Autodesk Fusion 360 part; units mm, degrees
(part 3 of 5)
sketch "Rack Tooth" plane through (0, 7, 0) normal (0, 1, 0) x (-1, 0, 0)
  line L0 (-33, 45.0877) -> (-33, 8.0877) construction
  circle A0 centre (-25, 30) radius 8 construction
  line L1 (0, 30) -> (-50, 30) construction
  line L2 (-33, 30) -> (-27.4745, 14.8188) construction
  spline S0 degree 5 poles (-32.1641, 27.722) (-32.1682, 27.7207) (-32.1765, 27.7182) (-32.1891, 27.7148) (-32.206, 27.7109) (-32.2273, 27.707) (-32.2489, 27.7038) (-32.2705, 27.701) (-32.2923, 27.6984) (-32.3141, 27.696) (-32.3359, 27.6937) (-32.3578, 27.6917) (-32.3798, 27.6899) (-32.4018, 27.6885) (-32.4239, 27.6874) (-32.4461, 27.6866) (-32.4684, 27.686) (-32.4907, 27.6857) (-32.5131, 27.6856) (-32.5355, 27.6857) (-32.5579, 27.6859) (-32.5804, 27.6864) (-32.6029, 27.6871) (-32.6255, 27.6879) (-32.6481, 27.689) (-32.6708, 27.6903) (-32.6935, 27.6918) (-32.7162, 27.6934) (-32.7389, 27.6953) (-32.7617, 27.6973) (-32.7846, 27.6995) (-32.8074, 27.7018) (-32.8303, 27.7044) (-32.8532, 27.7071) (-32.8761, 27.71) (-32.8991, 27.713) (-32.9221, 27.7162) (-32.9451, 27.7196) (-32.9681, 27.7232) (-32.9912, 27.7269) (-33.0142, 27.7307) (-33.0373, 27.7348) (-33.0605, 27.7389) (-33.0836, 27.7433) (-33.1067, 27.7478) (-33.1299, 27.7524) (-33.1531, 27.7572) (-33.1763, 27.7622) (-33.1995, 27.7673) (-33.2227, 27.7725) (-33.246, 27.7779) (-33.2692, 27.7835) (-33.2925, 27.7892) (-33.3158, 27.795) (-33.3391, 27.801) (-33.3624, 27.8071) (-33.3857, 27.8134) (-33.409, 27.8198) (-33.4323, 27.8264) (-33.4557, 27.833) (-33.479, 27.8399) (-33.5023, 27.8469) (-33.5257, 27.854) (-33.549, 27.8612) (-33.5724, 27.8686) (-33.5958, 27.8762) (-33.6191, 27.8838) (-33.6425, 27.8916) (-33.6659, 27.8996) (-33.6892, 27.9076) (-33.7126, 27.9158) (-33.7313, 27.9225) (-33.7453, 27.9276) (-33.7547, 27.931) (-33.7594, 27.9327) knots 0 0 0 0 0 0 0.01428571 0.02857143 0.04285714 0.05714286 0.07142857 0.08571429 0.1 0.11428571 0.12857143 0.14285714 0.15714286 0.17142857 0.18571429 0.2 0.21428571 0.22857143 0.24285714 0.25714286 0.27142857 0.28571429 0.3 0.31428571 0.32857143 0.34285714 0.35714286 0.37142857 0.38571429 0.4 0.41428571 0.42857143 0.44285714 0.45714286 0.47142857 0.48571429 0.5 0.51428571 0.52857143 0.54285714 0.55714286 0.57142857 0.58571429 0.6 0.61428571 0.62857143 0.64285714 0.65714286 0.67142857 0.68571429 0.7 0.71428571 0.72857143 0.74285714 0.75714286 0.77142857 0.78571429 0.8 0.81428571 0.82857143 0.84285714 0.85714286 0.87142857 0.88571429 0.9 0.91428571 0.92857143 0.94285714 0.95714286 0.97142857 0.98571429 1 1 1 1 1 1
  line L3 (-31.8911, 27.8084) -> (-32.1641, 27.722)
  arc A1 (-31.2753, 27.5157) -> (-31.8911, 27.8084) centre (-31.7402, 27.3317) ccw
  circle A2 centre (-25, 30) radius 2.5
  arc A3 (-31.194, 32.6807) -> (-31.2753, 32.4843) centre (-25, 30) ccw
  arc A4 (-31.194, 32.6807) -> (-31.4224, 33.323) centre (-31.6529, 32.8793) ccw
  line L4 (-31.4224, 33.323) -> (-31.6766, 33.455)
  spline S1 degree 5 poles (-31.6766, 33.455) (-31.6804, 33.457) (-31.6881, 33.4611) (-31.6993, 33.4675) (-31.714, 33.4768) (-31.7319, 33.4891) (-31.7494, 33.5021) (-31.7667, 33.5154) (-31.7839, 33.5289) (-31.801, 33.5426) (-31.818, 33.5565) (-31.835, 33.5705) (-31.8518, 33.5848) (-31.8684, 33.5994) (-31.8848, 33.6142) (-31.9011, 33.6294) (-31.9172, 33.6447) (-31.9332, 33.6603) (-31.9491, 33.676) (-31.9649, 33.6919) (-31.9805, 33.708) (-31.9961, 33.7242) (-32.0116, 33.7406) (-32.0269, 33.7572) (-32.0421, 33.7739) (-32.0573, 33.7908) (-32.0723, 33.8079) (-32.0872, 33.8252) (-32.1019, 33.8426) (-32.1166, 33.8601) (-32.1312, 33.8778) (-32.1457, 33.8956) (-32.1601, 33.9136) (-32.1744, 33.9317) (-32.1886, 33.95) (-32.2026, 33.9684) (-32.2166, 33.9869) (-32.2305, 34.0056) (-32.2443, 34.0244) (-32.258, 34.0433) (-32.2715, 34.0623) (-32.285, 34.0815) (-32.2984, 34.1008) (-32.3117, 34.1202) (-32.3249, 34.1398) (-32.338, 34.1594) (-32.351, 34.1792) (-32.3639, 34.1991) (-32.3767, 34.2192) (-32.3894, 34.2393) (-32.402, 34.2595) (-32.4146, 34.2799) (-32.427, 34.3004) (-32.4393, 34.321) (-32.4516, 34.3417) (-32.4637, 34.3625) (-32.4757, 34.3834) (-32.4877, 34.4044) (-32.4996, 34.4256) (-32.5113, 34.4468) (-32.523, 34.4681) (-32.5346, 34.4896) (-32.546, 34.5111) (-32.5574, 34.5328) (-32.5687, 34.5545) (-32.5799, 34.5763) (-32.591, 34.5983) (-32.602, 34.6203) (-32.6129, 34.6425) (-32.6237, 34.6647) (-32.6345, 34.687) (-32.643, 34.705) (-32.6493, 34.7185) (-32.6535, 34.7275) (-32.6556, 34.732) knots 0 0 0 0 0 0 0.01428571 0.02857143 0.04285714 0.05714286 0.07142857 0.08571429 0.1 0.11428571 0.12857143 0.14285714 0.15714286 0.17142857 0.18571429 0.2 0.21428571 0.22857143 0.24285714 0.25714286 0.27142857 0.28571429 0.3 0.31428571 0.32857143 0.34285714 0.35714286 0.37142857 0.38571429 0.4 0.41428571 0.42857143 0.44285714 0.45714286 0.47142857 0.48571429 0.5 0.51428571 0.52857143 0.54285714 0.55714286 0.57142857 0.58571429 0.6 0.61428571 0.62857143 0.64285714 0.65714286 0.67142857 0.68571429 0.7 0.71428571 0.72857143 0.74285714 0.75714286 0.77142857 0.78571429 0.8 0.81428571 0.82857143 0.84285714 0.85714286 0.87142857 0.88571429 0.9 0.91428571 0.92857143 0.94285714 0.95714286 0.97142857 0.98571429 1 1 1 1 1 1
  arc A5 (-32.3015, 35.262) -> (-32.6556, 34.732) centre (-25, 30) ccw
  spline S2 degree 5 poles (-30.747, 34.8462) (-30.7503, 34.849) (-30.757, 34.8545) (-30.7673, 34.8624) (-30.7814, 34.8724) (-30.7997, 34.8842) (-30.8184, 34.8954) (-30.8373, 34.9063) (-30.8564, 34.917) (-30.8756, 34.9276) (-30.8949, 34.938) (-30.9144, 34.9483) (-30.934, 34.9583) (-30.9538, 34.9681) (-30.9738, 34.9776) (-30.994, 34.9868) (-31.0144, 34.9959) (-31.0349, 35.0047) (-31.0555, 35.0133) (-31.0762, 35.0218) (-31.0971, 35.0302) (-31.118, 35.0384) (-31.1391, 35.0464) (-31.1603, 35.0542) (-31.1816, 35.0619) (-31.203, 35.0694) (-31.2245, 35.0767) (-31.2461, 35.0838) (-31.2679, 35.0909) (-31.2897, 35.0977) (-31.3116, 35.1044) (-31.3336, 35.111) (-31.3557, 35.1174) (-31.3779, 35.1237) (-31.4002, 35.1298) (-31.4226, 35.1357) (-31.4451, 35.1416) (-31.4676, 35.1472) (-31.4903, 35.1528) (-31.513, 35.1582) (-31.5358, 35.1634) (-31.5587, 35.1686) (-31.5816, 35.1735) (-31.6047, 35.1784) (-31.6278, 35.1831) (-31.651, 35.1877) (-31.6742, 35.1921) (-31.6975, 35.1964) (-31.7209, 35.2006) (-31.7444, 35.2046) (-31.7679, 35.2085) (-31.7916, 35.2123) (-31.8152, 35.216) (-31.839, 35.2195) (-31.8628, 35.2229) (-31.8866, 35.2261) (-31.9106, 35.2292) (-31.9346, 35.2322) (-31.9586, 35.2351) (-31.9828, 35.2378) (-32.0069, 35.2405) (-32.0312, 35.2429) (-32.0555, 35.2453) (-32.0798, 35.2475) (-32.1042, 35.2497) (-32.1287, 35.2516) (-32.1532, 35.2535) (-32.1778, 35.2552) (-32.2024, 35.2568) (-32.2271, 35.2583) (-32.2518, 35.2597) (-32.2717, 35.2607) (-32.2865, 35.2614) (-32.2965, 35.2618) (-32.3015, 35.262) knots 0 0 0 0 0 0 0.01428571 0.02857143 0.04285714 0.05714286 0.07142857 0.08571429 0.1 0.11428571 0.12857143 0.14285714 0.15714286 0.17142857 0.18571429 0.2 0.21428571 0.22857143 0.24285714 0.25714286 0.27142857 0.28571429 0.3 0.31428571 0.32857143 0.34285714 0.35714286 0.37142857 0.38571429 0.4 0.41428571 0.42857143 0.44285714 0.45714286 0.47142857 0.48571429 0.5 0.51428571 0.52857143 0.54285714 0.55714286 0.57142857 0.58571429 0.6 0.61428571 0.62857143 0.64285714 0.65714286 0.67142857 0.68571429 0.7 0.71428571 0.72857143 0.74285714 0.75714286 0.77142857 0.78571429 0.8 0.81428571 0.82857143 0.84285714 0.85714286 0.87142857 0.88571429 0.9 0.91428571 0.92857143 0.94285714 0.95714286 0.97142857 0.98571429 1 1 1 1 1 1
  line L5 (-30.747, 34.8462) -> (-30.5278, 34.6619)
  arc A6 (-30.5278, 34.6619) -> (-29.847, 34.6967) centre (-30.206, 35.0446) ccw
  arc A7 (-29.6967, 34.847) -> (-29.847, 34.6967) centre (-25, 30) ccw
  arc A8 (-29.6967, 34.847) -> (-29.6619, 35.5278) centre (-30.0446, 35.206) ccw
  line L6 (-29.6619, 35.5278) -> (-29.8462, 35.747)
  spline S3 degree 5 poles (-29.8462, 35.747) (-29.849, 35.7503) (-29.8545, 35.757) (-29.8624, 35.7673) (-29.8724, 35.7814) (-29.8842, 35.7997) (-29.8954, 35.8184) (-29.9063, 35.8373) (-29.917, 35.8564) (-29.9276, 35.8756) (-29.938, 35.8949) (-29.9483, 35.9144) (-29.9583, 35.934) (-29.9681, 35.9538) (-29.9776, 35.9738) (-29.9868, 35.994) (-29.9959, 36.0144) (-30.0047, 36.0349) (-30.0133, 36.0555) (-30.0218, 36.0762) (-30.0302, 36.0971) (-30.0384, 36.118) (-30.0464, 36.1391) (-30.0542, 36.1603) (-30.0619, 36.1816) (-30.0694, 36.203) (-30.0767, 36.2245) (-30.0838, 36.2461) (-30.0909, 36.2679) (-30.0977, 36.2897) (-30.1044, 36.3116) (-30.111, 36.3336) (-30.1174, 36.3557) (-30.1237, 36.3779) (-30.1298, 36.4002) (-30.1357, 36.4226) (-30.1416, 36.4451) (-30.1472, 36.4676) (-30.1528, 36.4903) (-30.1582, 36.513) (-30.1634, 36.5358) (-30.1686, 36.5587) (-30.1735, 36.5816) (-30.1784, 36.6047) (-30.1831, 36.6278) (-30.1877, 36.651) (-30.1921, 36.6742) (-30.1964, 36.6975) (-30.2006, 36.7209) (-30.2046, 36.7444) (-30.2085, 36.7679) (-30.2123, 36.7916) (-30.216, 36.8152) (-30.2195, 36.839) (-30.2229, 36.8628) (-30.2261, 36.8866) (-30.2292, 36.9106) (-30.2322, 36.9346) (-30.2351, 36.9586) (-30.2378, 36.9828) (-30.2405, 37.0069) (-30.2429, 37.0312) (-30.2453, 37.0555) (-30.2475, 37.0798) (-30.2497, 37.1042) (-30.2516, 37.1287) (-30.2535, 37.1532) (-30.2552, 37.1778) (-30.2568, 37.2024) (-30.2583, 37.2271) (-30.2597, 37.2518) (-30.2607, 37.2717) (-30.2614, 37.2865) (-30.2618, 37.2965) (-30.262, 37.3015) knots 0 0 0 0 0 0 0.01428571 0.02857143 0.04285714 0.05714286 0.07142857 0.08571429 0.1 0.11428571 0.12857143 0.14285714 0.15714286 0.17142857 0.18571429 0.2 0.21428571 0.22857143 0.24285714 0.25714286 0.27142857 0.28571429 0.3 0.31428571 0.32857143 0.34285714 0.35714286 0.37142857 0.38571429 0.4 0.41428571 0.42857143 0.44285714 0.45714286 0.47142857 0.48571429 0.5 0.51428571 0.52857143 0.54285714 0.55714286 0.57142857 0.58571429 0.6 0.61428571 0.62857143 0.64285714 0.65714286 0.67142857 0.68571429 0.7 0.71428571 0.72857143 0.74285714 0.75714286 0.77142857 0.78571429 0.8 0.81428571 0.82857143 0.84285714 0.85714286 0.87142857 0.88571429 0.9 0.91428571 0.92857143 0.94285714 0.95714286 0.97142857 0.98571429 1 1 1 1 1 1
  arc A9 (-29.732, 37.6556) -> (-30.262, 37.3015) centre (-25, 30) ccw
  spline S4 degree 5 poles (-28.455, 36.6766) (-28.457, 36.6804) (-28.4611, 36.6881) (-28.4675, 36.6993) (-28.4768, 36.714) (-28.4891, 36.7319) (-28.5021, 36.7494) (-28.5154, 36.7667) (-28.5289, 36.7839) (-28.5426, 36.801) (-28.5565, 36.818) (-28.5705, 36.835) (-28.5848, 36.8518) (-28.5994, 36.8684) (-28.6142, 36.8848) (-28.6294, 36.9011) (-28.6447, 36.9172) (-28.6603, 36.9332) (-28.676, 36.9491) (-28.6919, 36.9649) (-28.708, 36.9805) (-28.7242, 36.9961) (-28.7406, 37.0116) (-28.7572, 37.0269) (-28.7739, 37.0421) (-28.7908, 37.0573) (-28.8079, 37.0723) (-28.8252, 37.0872) (-28.8426, 37.1019) (-28.8601, 37.1166) (-28.8778, 37.1312) (-28.8956, 37.1457) (-28.9136, 37.1601) (-28.9317, 37.1744) (-28.95, 37.1886) (-28.9684, 37.2026) (-28.9869, 37.2166) (-29.0056, 37.2305) (-29.0244, 37.2443) (-29.0433, 37.258) (-29.0623, 37.2715) (-29.0815, 37.285) (-29.1008, 37.2984) (-29.1202, 37.3117) (-29.1398, 37.3249) (-29.1594, 37.338) (-29.1792, 37.351) (-29.1991, 37.3639) (-29.2192, 37.3767) (-29.2393, 37.3894) (-29.2595, 37.402) (-29.2799, 37.4146) (-29.3004, 37.427) (-29.321, 37.4393) (-29.3417, 37.4516) (-29.3625, 37.4637) (-29.3834, 37.4757) (-29.4044, 37.4877) (-29.4256, 37.4996) (-29.4468, 37.5113) (-29.4681, 37.523) (-29.4896, 37.5346) (-29.5111, 37.546) (-29.5328, 37.5574) (-29.5545, 37.5687) (-29.5763, 37.5799) (-29.5983, 37.591) (-29.6203, 37.602) (-29.6425, 37.6129) (-29.6647, 37.6237) (-29.687, 37.6345) (-29.705, 37.643) (-29.7185, 37.6493) (-29.7275, 37.6535) (-29.732, 37.6556) knots 0 0 0 0 0 0 0.01428571 0.02857143 0.04285714 0.05714286 0.07142857 0.08571429 0.1 0.11428571 0.12857143 0.14285714 0.15714286 0.17142857 0.18571429 0.2 0.21428571 0.22857143 0.24285714 0.25714286 0.27142857 0.28571429 0.3 0.31428571 0.32857143 0.34285714 0.35714286 0.37142857 0.38571429 0.4 0.41428571 0.42857143 0.44285714 0.45714286 0.47142857 0.48571429 0.5 0.51428571 0.52857143 0.54285714 0.55714286 0.57142857 0.58571429 0.6 0.61428571 0.62857143 0.64285714 0.65714286 0.67142857 0.68571429 0.7 0.71428571 0.72857143 0.74285714 0.75714286 0.77142857 0.78571429 0.8 0.81428571 0.82857143 0.84285714 0.85714286 0.87142857 0.88571429 0.9 0.91428571 0.92857143 0.94285714 0.95714286 0.97142857 0.98571429 1 1 1 1 1 1
  line L7 (-28.455, 36.6766) -> (-28.323, 36.4224)
  arc A10 (-28.323, 36.4224) -> (-27.6807, 36.194) centre (-27.8793, 36.6529) ccw
  arc A11 (-27.4843, 36.2753) -> (-27.6807, 36.194) centre (-25, 30) ccw
  arc A12 (-27.4843, 36.2753) -> (-27.1916, 36.8911) centre (-27.6683, 36.7402) ccw
  line L8 (-27.1916, 36.8911) -> (-27.278, 37.1641)
  spline S5 degree 5 poles (-27.278, 37.1641) (-27.2793, 37.1682) (-27.2818, 37.1765) (-27.2852, 37.1891) (-27.2891, 37.206) (-27.293, 37.2273) (-27.2962, 37.2489) (-27.299, 37.2705) (-27.3016, 37.2923) (-27.304, 37.3141) (-27.3063, 37.3359) (-27.3083, 37.3578) (-27.3101, 37.3798) (-27.3115, 37.4018) (-27.3126, 37.4239) (-27.3134, 37.4461) (-27.314, 37.4684) (-27.3143, 37.4907) (-27.3144, 37.5131) (-27.3143, 37.5355) (-27.3141, 37.5579) (-27.3136, 37.5804) (-27.3129, 37.6029) (-27.3121, 37.6255) (-27.311, 37.6481) (-27.3097, 37.6708) (-27.3082, 37.6935) (-27.3066, 37.7162) (-27.3047, 37.7389) (-27.3027, 37.7617) (-27.3005, 37.7846) (-27.2982, 37.8074) (-27.2956, 37.8303) (-27.2929, 37.8532) (-27.29, 37.8761) (-27.287, 37.8991) (-27.2838, 37.9221) (-27.2804, 37.9451) (-27.2768, 37.9681) (-27.2731, 37.9912) (-27.2693, 38.0142) (-27.2652, 38.0373) (-27.2611, 38.0605) (-27.2567, 38.0836) (-27.2522, 38.1067) (-27.2476, 38.1299) (-27.2428, 38.1531) (-27.2378, 38.1763) (-27.2327, 38.1995) (-27.2275, 38.2227) (-27.2221, 38.246) (-27.2165, 38.2692) (-27.2108, 38.2925) (-27.205, 38.3158) (-27.199, 38.3391) (-27.1929, 38.3624) (-27.1866, 38.3857) (-27.1802, 38.409) (-27.1736, 38.4323) (-27.167, 38.4557) (-27.1601, 38.479) (-27.1531, 38.5023) (-27.146, 38.5257) (-27.1388, 38.549) (-27.1314, 38.5724) (-27.1238, 38.5958) (-27.1162, 38.6191) (-27.1084, 38.6425) (-27.1004, 38.6659) (-27.0924, 38.6892) (-27.0842, 38.7126) (-27.0775, 38.7313) (-27.0724, 38.7453) (-27.069, 38.7547) (-27.0673, 38.7594) knots 0 0 0 0 0 0 0.01428571 0.02857143 0.04285714 0.05714286 0.07142857 0.08571429 0.1 0.11428571 0.12857143 0.14285714 0.15714286 0.17142857 0.18571429 0.2 0.21428571 0.22857143 0.24285714 0.25714286 0.27142857 0.28571429 0.3 0.31428571 0.32857143 0.34285714 0.35714286 0.37142857 0.38571429 0.4 0.41428571 0.42857143 0.44285714 0.45714286 0.47142857 0.48571429 0.5 0.51428571 0.52857143 0.54285714 0.55714286 0.57142857 0.58571429 0.6 0.61428571 0.62857143 0.64285714 0.65714286 0.67142857 0.68571429 0.7 0.71428571 0.72857143 0.74285714 0.75714286 0.77142857 0.78571429 0.8 0.81428571 0.82857143 0.84285714 0.85714286 0.87142857 0.88571429 0.9 0.91428571 0.92857143 0.94285714 0.95714286 0.97142857 0.98571429 1 1 1 1 1 1
  arc A13 (-26.4421, 38.8837) -> (-27.0673, 38.7594) centre (-25, 30) ccw
  spline S6 degree 5 poles (-25.637, 37.4905) (-25.6373, 37.4948) (-25.6382, 37.5035) (-25.6399, 37.5163) (-25.6428, 37.5334) (-25.6473, 37.5547) (-25.6526, 37.5758) (-25.6583, 37.5969) (-25.6642, 37.618) (-25.6703, 37.639) (-25.6766, 37.6601) (-25.6831, 37.6811) (-25.6899, 37.702) (-25.697, 37.723) (-25.7044, 37.7438) (-25.7122, 37.7646) (-25.7202, 37.7854) (-25.7285, 37.8061) (-25.7369, 37.8269) (-25.7456, 37.8475) (-25.7544, 37.8682) (-25.7634, 37.8888) (-25.7726, 37.9093) (-25.7821, 37.9298) (-25.7917, 37.9503) (-25.8016, 37.9707) (-25.8116, 37.9911) (-25.8219, 38.0115) (-25.8323, 38.0318) (-25.8429, 38.0521) (-25.8536, 38.0724) (-25.8645, 38.0926) (-25.8756, 38.1127) (-25.8869, 38.1329) (-25.8984, 38.1529) (-25.91, 38.173) (-25.9217, 38.193) (-25.9337, 38.213) (-25.9458, 38.2329) (-25.958, 38.2528) (-25.9704, 38.2726) (-25.983, 38.2924) (-25.9957, 38.3122) (-26.0085, 38.3319) (-26.0215, 38.3515) (-26.0347, 38.3712) (-26.048, 38.3908) (-26.0615, 38.4103) (-26.075, 38.4298) (-26.0888, 38.4492) (-26.1027, 38.4687) (-26.1167, 38.488) (-26.1309, 38.5073) (-26.1452, 38.5266) (-26.1596, 38.5458) (-26.1742, 38.565) (-26.1889, 38.5841) (-26.2037, 38.6032) (-26.2187, 38.6223) (-26.2338, 38.6413) (-26.2491, 38.6602) (-26.2645, 38.6791) (-26.28, 38.698) (-26.2956, 38.7168) (-26.3114, 38.7355) (-26.3273, 38.7542) (-26.3433, 38.7729) (-26.3595, 38.7915) (-26.3757, 38.81) (-26.3921, 38.8285) (-26.4087, 38.847) (-26.422, 38.8617) (-26.432, 38.8727) (-26.4387, 38.88) (-26.4421, 38.8837) knots 0 0 0 0 0 0 0.01428571 0.02857143 0.04285714 0.05714286 0.07142857 0.08571429 0.1 0.11428571 0.12857143 0.14285714 0.15714286 0.17142857 0.18571429 0.2 0.21428571 0.22857143 0.24285714 0.25714286 0.27142857 0.28571429 0.3 0.31428571 0.32857143 0.34285714 0.35714286 0.37142857 0.38571429 0.4 0.41428571 0.42857143 0.44285714 0.45714286 0.47142857 0.48571429 0.5 0.51428571 0.52857143 0.54285714 0.55714286 0.57142857 0.58571429 0.6 0.61428571 0.62857143 0.64285714 0.65714286 0.67142857 0.68571429 0.7 0.71428571 0.72857143 0.74285714 0.75714286 0.77142857 0.78571429 0.8 0.81428571 0.82857143 0.84285714 0.85714286 0.87142857 0.88571429 0.9 0.91428571 0.92857143 0.94285714 0.95714286 0.97142857 0.98571429 1 1 1 1 1 1
  line L9 (-25.637, 37.4905) -> (-25.6123, 37.2052)
  arc A14 (-25.6123, 37.2052) -> (-25.1063, 36.7484) centre (-25.1142, 37.2483) ccw
  arc A15 (-24.8937, 36.7484) -> (-25.1063, 36.7484) centre (-25, 30) ccw
  arc A16 (-24.8937, 36.7484) -> (-24.3877, 37.2052) centre (-24.8858, 37.2483) ccw
  line L10 (-24.3877, 37.2052) -> (-24.363, 37.4905)
  spline S7 degree 5 poles (-24.363, 37.4905) (-24.3627, 37.4948) (-24.3618, 37.5035) (-24.3601, 37.5163) (-24.3572, 37.5334) (-24.3527, 37.5547) (-24.3474, 37.5758) (-24.3417, 37.5969) (-24.3358, 37.618) (-24.3297, 37.639) (-24.3234, 37.6601) (-24.3169, 37.6811) (-24.3101, 37.702) (-24.303, 37.723) (-24.2956, 37.7438) (-24.2878, 37.7646) (-24.2798, 37.7854) (-24.2715, 37.8061) (-24.2631, 37.8269) (-24.2544, 37.8475) (-24.2456, 37.8682) (-24.2366, 37.8888) (-24.2274, 37.9093) (-24.2179, 37.9298) (-24.2083, 37.9503) (-24.1984, 37.9707) (-24.1884, 37.9911) (-24.1781, 38.0115) (-24.1677, 38.0318) (-24.1571, 38.0521) (-24.1464, 38.0724) (-24.1355, 38.0926) (-24.1244, 38.1127) (-24.1131, 38.1329) (-24.1016, 38.1529) (-24.09, 38.173) (-24.0783, 38.193) (-24.0663, 38.213) (-24.0542, 38.2329) (-24.042, 38.2528) (-24.0296, 38.2726) (-24.017, 38.2924) (-24.0043, 38.3122) (-23.9915, 38.3319) (-23.9785, 38.3515) (-23.9653, 38.3712) (-23.952, 38.3908) (-23.9385, 38.4103) (-23.925, 38.4298) (-23.9112, 38.4492) (-23.8973, 38.4687) (-23.8833, 38.488) (-23.8691, 38.5073) (-23.8548, 38.5266) (-23.8404, 38.5458) (-23.8258, 38.565) (-23.8111, 38.5841) (-23.7963, 38.6032) (-23.7813, 38.6223) (-23.7662, 38.6413) (-23.7509, 38.6602) (-23.7355, 38.6791) (-23.72, 38.698) (-23.7044, 38.7168) (-23.6886, 38.7355) (-23.6727, 38.7542) (-23.6567, 38.7729) (-23.6405, 38.7915) (-23.6243, 38.81) (-23.6079, 38.8285) (-23.5913, 38.847) (-23.578, 38.8617) (-23.568, 38.8727) (-23.5613, 38.88) (-23.5579, 38.8837) knots 0 0 0 0 0 0 0.01428571 0.02857143 0.04285714 0.05714286 0.07142857 0.08571429 0.1 0.11428571 0.12857143 0.14285714 0.15714286 0.17142857 0.18571429 0.2 0.21428571 0.22857143 0.24285714 0.25714286 0.27142857 0.28571429 0.3 0.31428571 0.32857143 0.34285714 0.35714286 0.37142857 0.38571429 0.4 0.41428571 0.42857143 0.44285714 0.45714286 0.47142857 0.48571429 0.5 0.51428571 0.52857143 0.54285714 0.55714286 0.57142857 0.58571429 0.6 0.61428571 0.62857143 0.64285714 0.65714286 0.67142857 0.68571429 0.7 0.71428571 0.72857143 0.74285714 0.75714286 0.77142857 0.78571429 0.8 0.81428571 0.82857143 0.84285714 0.85714286 0.87142857 0.88571429 0.9 0.91428571 0.92857143 0.94285714 0.95714286 0.97142857 0.98571429 1 1 1 1 1 1
  arc A17 (-22.9327, 38.7594) -> (-23.5579, 38.8837) centre (-25, 30) ccw
  spline S8 degree 5 poles (-22.722, 37.1641) (-22.7207, 37.1682) (-22.7182, 37.1765) (-22.7148, 37.1891) (-22.7109, 37.206) (-22.707, 37.2273) (-22.7038, 37.2489) (-22.701, 37.2705) (-22.6984, 37.2923) (-22.696, 37.3141) (-22.6937, 37.3359) (-22.6917, 37.3578) (-22.6899, 37.3798) (-22.6885, 37.4018) (-22.6874, 37.4239) (-22.6866, 37.4461) (-22.686, 37.4684) (-22.6857, 37.4907) (-22.6856, 37.5131) (-22.6857, 37.5355) (-22.6859, 37.5579) (-22.6864, 37.5804) (-22.6871, 37.6029) (-22.6879, 37.6255) (-22.689, 37.6481) (-22.6903, 37.6708) (-22.6918, 37.6935) (-22.6934, 37.7162) (-22.6953, 37.7389) (-22.6973, 37.7617) (-22.6995, 37.7846) (-22.7018, 37.8074) (-22.7044, 37.8303) (-22.7071, 37.8532) (-22.71, 37.8761) (-22.713, 37.8991) (-22.7162, 37.9221) (-22.7196, 37.9451) (-22.7232, 37.9681) (-22.7269, 37.9912) (-22.7307, 38.0142) (-22.7348, 38.0373) (-22.7389, 38.0605) (-22.7433, 38.0836) (-22.7478, 38.1067) (-22.7524, 38.1299) (-22.7572, 38.1531) (-22.7622, 38.1763) (-22.7673, 38.1995) (-22.7725, 38.2227) (-22.7779, 38.246) (-22.7835, 38.2692) (-22.7892, 38.2925) (-22.795, 38.3158) (-22.801, 38.3391) (-22.8071, 38.3624) (-22.8134, 38.3857) (-22.8198, 38.409) (-22.8264, 38.4323) (-22.833, 38.4557) (-22.8399, 38.479) (-22.8469, 38.5023) (-22.854, 38.5257) (-22.8612, 38.549) (-22.8686, 38.5724) (-22.8762, 38.5958) (-22.8838, 38.6191) (-22.8916, 38.6425) (-22.8996, 38.6659) (-22.9076, 38.6892) (-22.9158, 38.7126) (-22.9225, 38.7313) (-22.9276, 38.7453) (-22.931, 38.7547) (-22.9327, 38.7594) knots 0 0 0 0 0 0 0.01428571 0.02857143 0.04285714 0.05714286 0.07142857 0.08571429 0.1 0.11428571 0.12857143 0.14285714 0.15714286 0.17142857 0.18571429 0.2 0.21428571 0.22857143 0.24285714 0.25714286 0.27142857 0.28571429 0.3 0.31428571 0.32857143 0.34285714 0.35714286 0.37142857 0.38571429 0.4 0.41428571 0.42857143 0.44285714 0.45714286 0.47142857 0.48571429 0.5 0.51428571 0.52857143 0.54285714 0.55714286 0.57142857 0.58571429 0.6 0.61428571 0.62857143 0.64285714 0.65714286 0.67142857 0.68571429 0.7 0.71428571 0.72857143 0.74285714 0.75714286 0.77142857 0.78571429 0.8 0.81428571 0.82857143 0.84285714 0.85714286 0.87142857 0.88571429 0.9 0.91428571 0.92857143 0.94285714 0.95714286 0.97142857 0.98571429 1 1 1 1 1 1
  line L11 (-22.722, 37.1641) -> (-22.8084, 36.8911)
  arc A18 (-22.8084, 36.8911) -> (-22.5157, 36.2753) centre (-22.3317, 36.7402) ccw
  arc A19 (-22.3193, 36.194) -> (-22.5157, 36.2753) centre (-25, 30) ccw
  arc A20 (-22.3193, 36.194) -> (-21.677, 36.4224) centre (-22.1207, 36.6529) ccw
  line L12 (-21.677, 36.4224) -> (-21.545, 36.6766)
  spline S9 degree 5 poles (-21.545, 36.6766) (-21.543, 36.6804) (-21.5389, 36.6881) (-21.5325, 36.6993) (-21.5232, 36.714) (-21.5109, 36.7319) (-21.4979, 36.7494) (-21.4846, 36.7667) (-21.4711, 36.7839) (-21.4574, 36.801) (-21.4435, 36.818) (-21.4295, 36.835) (-21.4152, 36.8518) (-21.4006, 36.8684) (-21.3858, 36.8848) (-21.3706, 36.9011) (-21.3553, 36.9172) (-21.3397, 36.9332) (-21.324, 36.9491) (-21.3081, 36.9649) (-21.292, 36.9805) (-21.2758, 36.9961) (-21.2594, 37.0116) (-21.2428, 37.0269) (-21.2261, 37.0421) (-21.2092, 37.0573) (-21.1921, 37.0723) (-21.1748, 37.0872) (-21.1574, 37.1019) (-21.1399, 37.1166) (-21.1222, 37.1312) (-21.1044, 37.1457) (-21.0864, 37.1601) (-21.0683, 37.1744) (-21.05, 37.1886) (-21.0316, 37.2026) (-21.0131, 37.2166) (-20.9944, 37.2305) (-20.9756, 37.2443) (-20.9567, 37.258) (-20.9377, 37.2715) (-20.9185, 37.285) (-20.8992, 37.2984) (-20.8798, 37.3117) (-20.8602, 37.3249) (-20.8406, 37.338) (-20.8208, 37.351) (-20.8009, 37.3639) (-20.7808, 37.3767) (-20.7607, 37.3894) (-20.7405, 37.402) (-20.7201, 37.4146) (-20.6996, 37.427) (-20.679, 37.4393) (-20.6583, 37.4516) (-20.6375, 37.4637) (-20.6166, 37.4757) (-20.5956, 37.4877) (-20.5744, 37.4996) (-20.5532, 37.5113) (-20.5319, 37.523) (-20.5104, 37.5346) (-20.4889, 37.546) (-20.4672, 37.5574) (-20.4455, 37.5687) (-20.4237, 37.5799) (-20.4017, 37.591) (-20.3797, 37.602) (-20.3575, 37.6129) (-20.3353, 37.6237) (-20.313, 37.6345) (-20.295, 37.643) (-20.2815, 37.6493) (-20.2725, 37.6535) (-20.268, 37.6556) knots 0 0 0 0 0 0 0.01428571 0.02857143 0.04285714 0.05714286 0.07142857 0.08571429 0.1 0.11428571 0.12857143 0.14285714 0.15714286 0.17142857 0.18571429 0.2 0.21428571 0.22857143 0.24285714 0.25714286 0.27142857 0.28571429 0.3 0.31428571 0.32857143 0.34285714 0.35714286 0.37142857 0.38571429 0.4 0.41428571 0.42857143 0.44285714 0.45714286 0.47142857 0.48571429 0.5 0.51428571 0.52857143 0.54285714 0.55714286 0.57142857 0.58571429 0.6 0.61428571 0.62857143 0.64285714 0.65714286 0.67142857 0.68571429 0.7 0.71428571 0.72857143 0.74285714 0.75714286 0.77142857 0.78571429 0.8 0.81428571 0.82857143 0.84285714 0.85714286 0.87142857 0.88571429 0.9 0.91428571 0.92857143 0.94285714 0.95714286 0.97142857 0.98571429 1 1 1 1 1 1
  arc A21 (-19.738, 37.3015) -> (-20.268, 37.6556) centre (-25, 30) ccw
  spline S10 degree 5 poles (-20.1538, 35.747) (-20.151, 35.7503) (-20.1455, 35.757) (-20.1376, 35.7673) (-20.1276, 35.7814) (-20.1158, 35.7997) (-20.1046, 35.8184) (-20.0937, 35.8373) (-20.083, 35.8564) (-20.0724, 35.8756) (-20.062, 35.8949) (-20.0517, 35.9144) (-20.0417, 35.934) (-20.0319, 35.9538) (-20.0224, 35.9738) (-20.0132, 35.994) (-20.0041, 36.0144) (-19.9953, 36.0349) (-19.9867, 36.0555) (-19.9782, 36.0762) (-19.9698, 36.0971) (-19.9616, 36.118) (-19.9536, 36.1391) (-19.9458, 36.1603) (-19.9381, 36.1816) (-19.9306, 36.203) (-19.9233, 36.2245) (-19.9162, 36.2461) (-19.9091, 36.2679) (-19.9023, 36.2897) (-19.8956, 36.3116) (-19.889, 36.3336) (-19.8826, 36.3557) (-19.8763, 36.3779) (-19.8702, 36.4002) (-19.8643, 36.4226) (-19.8584, 36.4451) (-19.8528, 36.4676) (-19.8472, 36.4903) (-19.8418, 36.513) (-19.8366, 36.5358) (-19.8314, 36.5587) (-19.8265, 36.5816) (-19.8216, 36.6047) (-19.8169, 36.6278) (-19.8123, 36.651) (-19.8079, 36.6742) (-19.8036, 36.6975) (-19.7994, 36.7209) (-19.7954, 36.7444) (-19.7915, 36.7679) (-19.7877, 36.7916) (-19.784, 36.8152) (-19.7805, 36.839) (-19.7771, 36.8628) (-19.7739, 36.8866) (-19.7708, 36.9106) (-19.7678, 36.9346) (-19.7649, 36.9586) (-19.7622, 36.9828) (-19.7595, 37.0069) (-19.7571, 37.0312) (-19.7547, 37.0555) (-19.7525, 37.0798) (-19.7503, 37.1042) (-19.7484, 37.1287) (-19.7465, 37.1532) (-19.7448, 37.1778) (-19.7432, 37.2024) (-19.7417, 37.2271) (-19.7403, 37.2518) (-19.7393, 37.2717) (-19.7386, 37.2865) (-19.7382, 37.2965) (-19.738, 37.3015) knots 0 0 0 0 0 0 0.01428571 0.02857143 0.04285714 0.05714286 0.07142857 0.08571429 0.1 0.11428571 0.12857143 0.14285714 0.15714286 0.17142857 0.18571429 0.2 0.21428571 0.22857143 0.24285714 0.25714286 0.27142857 0.28571429 0.3 0.31428571 0.32857143 0.34285714 0.35714286 0.37142857 0.38571429 0.4 0.41428571 0.42857143 0.44285714 0.45714286 0.47142857 0.48571429 0.5 0.51428571 0.52857143 0.54285714 0.55714286 0.57142857 0.58571429 0.6 0.61428571 0.62857143 0.64285714 0.65714286 0.67142857 0.68571429 0.7 0.71428571 0.72857143 0.74285714 0.75714286 0.77142857 0.78571429 0.8 0.81428571 0.82857143 0.84285714 0.85714286 0.87142857 0.88571429 0.9 0.91428571 0.92857143 0.94285714 0.95714286 0.97142857 0.98571429 1 1 1 1 1 1
  line L13 (-20.1538, 35.747) -> (-20.3381, 35.5278)
  arc A22 (-20.3381, 35.5278) -> (-20.3033, 34.847) centre (-19.9554, 35.206) ccw
  arc A23 (-20.153, 34.6967) -> (-20.3033, 34.847) centre (-25, 30) ccw
  arc A24 (-20.153, 34.6967) -> (-19.4722, 34.6619) centre (-19.794, 35.0446) ccw
  line L14 (-19.4722, 34.6619) -> (-19.253, 34.8462)
  spline S11 degree 5 poles (-19.253, 34.8462) (-19.2497, 34.849) (-19.243, 34.8545) (-19.2327, 34.8624) (-19.2186, 34.8724) (-19.2003, 34.8842) (-19.1816, 34.8954) (-19.1627, 34.9063) (-19.1436, 34.917) (-19.1244, 34.9276) (-19.1051, 34.938) (-19.0856, 34.9483) (-19.066, 34.9583) (-19.0462, 34.9681) (-19.0262, 34.9776) (-19.006, 34.9868) (-18.9856, 34.9959) (-18.9651, 35.0047) (-18.9445, 35.0133) (-18.9238, 35.0218) (-18.9029, 35.0302) (-18.882, 35.0384) (-18.8609, 35.0464) (-18.8397, 35.0542) (-18.8184, 35.0619) (-18.797, 35.0694) (-18.7755, 35.0767) (-18.7539, 35.0838) (-18.7321, 35.0909) (-18.7103, 35.0977) (-18.6884, 35.1044) (-18.6664, 35.111) (-18.6443, 35.1174) (-18.6221, 35.1237) (-18.5998, 35.1298) (-18.5774, 35.1357) (-18.5549, 35.1416) (-18.5324, 35.1472) (-18.5097, 35.1528) (-18.487, 35.1582) (-18.4642, 35.1634) (-18.4413, 35.1686) (-18.4184, 35.1735) (-18.3953, 35.1784) (-18.3722, 35.1831) (-18.349, 35.1877) (-18.3258, 35.1921) (-18.3025, 35.1964) (-18.2791, 35.2006) (-18.2556, 35.2046) (-18.2321, 35.2085) (-18.2084, 35.2123) (-18.1848, 35.216) (-18.161, 35.2195) (-18.1372, 35.2229) (-18.1134, 35.2261) (-18.0894, 35.2292) (-18.0654, 35.2322) (-18.0414, 35.2351) (-18.0172, 35.2378) (-17.9931, 35.2405) (-17.9688, 35.2429) (-17.9445, 35.2453) (-17.9202, 35.2475) (-17.8958, 35.2497) (-17.8713, 35.2516) (-17.8468, 35.2535) (-17.8222, 35.2552) (-17.7976, 35.2568) (-17.7729, 35.2583) (-17.7482, 35.2597) (-17.7283, 35.2607) (-17.7135, 35.2614) (-17.7035, 35.2618) (-17.6985, 35.262) knots 0 0 0 0 0 0 0.01428571 0.02857143 0.04285714 0.05714286 0.07142857 0.08571429 0.1 0.11428571 0.12857143 0.14285714 0.15714286 0.17142857 0.18571429 0.2 0.21428571 0.22857143 0.24285714 0.25714286 0.27142857 0.28571429 0.3 0.31428571 0.32857143 0.34285714 0.35714286 0.37142857 0.38571429 0.4 0.41428571 0.42857143 0.44285714 0.45714286 0.47142857 0.48571429 0.5 0.51428571 0.52857143 0.54285714 0.55714286 0.57142857 0.58571429 0.6 0.61428571 0.62857143 0.64285714 0.65714286 0.67142857 0.68571429 0.7 0.71428571 0.72857143 0.74285714 0.75714286 0.77142857 0.78571429 0.8 0.81428571 0.82857143 0.84285714 0.85714286 0.87142857 0.88571429 0.9 0.91428571 0.92857143 0.94285714 0.95714286 0.97142857 0.98571429 1 1 1 1 1 1
  arc A25 (-17.3444, 34.732) -> (-17.6985, 35.262) centre (-25, 30) ccw
  spline S12 degree 5 poles (-18.3234, 33.455) (-18.3196, 33.457) (-18.3119, 33.4611) (-18.3007, 33.4675) (-18.286, 33.4768) (-18.2681, 33.4891) (-18.2506, 33.5021) (-18.2333, 33.5154) (-18.2161, 33.5289) (-18.199, 33.5426) (-18.182, 33.5565) (-18.165, 33.5705) (-18.1482, 33.5848) (-18.1316, 33.5994) (-18.1152, 33.6142) (-18.0989, 33.6294) (-18.0828, 33.6447) (-18.0668, 33.6603) (-18.0509, 33.676) (-18.0351, 33.6919) (-18.0195, 33.708) (-18.0039, 33.7242) (-17.9884, 33.7406) (-17.9731, 33.7572) (-17.9579, 33.7739) (-17.9427, 33.7908) (-17.9277, 33.8079) (-17.9128, 33.8252) (-17.8981, 33.8426) (-17.8834, 33.8601) (-17.8688, 33.8778) (-17.8543, 33.8956) (-17.8399, 33.9136) (-17.8256, 33.9317) (-17.8114, 33.95) (-17.7974, 33.9684) (-17.7834, 33.9869) (-17.7695, 34.0056) (-17.7557, 34.0244) (-17.742, 34.0433) (-17.7285, 34.0623) (-17.715, 34.0815) (-17.7016, 34.1008) (-17.6883, 34.1202) (-17.6751, 34.1398) (-17.662, 34.1594) (-17.649, 34.1792) (-17.6361, 34.1991) (-17.6233, 34.2192) (-17.6106, 34.2393) (-17.598, 34.2595) (-17.5854, 34.2799) (-17.573, 34.3004) (-17.5607, 34.321) (-17.5484, 34.3417) (-17.5363, 34.3625) (-17.5243, 34.3834) (-17.5123, 34.4044) (-17.5004, 34.4256) (-17.4887, 34.4468) (-17.477, 34.4681) (-17.4654, 34.4896) (-17.454, 34.5111) (-17.4426, 34.5328) (-17.4313, 34.5545) (-17.4201, 34.5763) (-17.409, 34.5983) (-17.398, 34.6203) (-17.3871, 34.6425) (-17.3763, 34.6647) (-17.3655, 34.687) (-17.357, 34.705) (-17.3507, 34.7185) (-17.3465, 34.7275) (-17.3444, 34.732) knots 0 0 0 0 0 0 0.01428571 0.02857143 0.04285714 0.05714286 0.07142857 0.08571429 0.1 0.11428571 0.12857143 0.14285714 0.15714286 0.17142857 0.18571429 0.2 0.21428571 0.22857143 0.24285714 0.25714286 0.27142857 0.28571429 0.3 0.31428571 0.32857143 0.34285714 0.35714286 0.37142857 0.38571429 0.4 0.41428571 0.42857143 0.44285714 0.45714286 0.47142857 0.48571429 0.5 0.51428571 0.52857143 0.54285714 0.55714286 0.57142857 0.58571429 0.6 0.61428571 0.62857143 0.64285714 0.65714286 0.67142857 0.68571429 0.7 0.71428571 0.72857143 0.74285714 0.75714286 0.77142857 0.78571429 0.8 0.81428571 0.82857143 0.84285714 0.85714286 0.87142857 0.88571429 0.9 0.91428571 0.92857143 0.94285714 0.95714286 0.97142857 0.98571429 1 1 1 1 1 1
  line L15 (-18.3234, 33.455) -> (-18.5776, 33.323)
  arc A26 (-18.5776, 33.323) -> (-18.806, 32.6807) centre (-18.3471, 32.8793) ccw
  arc A27 (-18.7247, 32.4843) -> (-18.806, 32.6807) centre (-25, 30) ccw
  arc A28 (-18.7247, 32.4843) -> (-18.1089, 32.1916) centre (-18.2598, 32.6683) ccw
  line L16 (-18.1089, 32.1916) -> (-17.8359, 32.278)
  spline S13 degree 5 poles (-17.8359, 32.278) (-17.8318, 32.2793) (-17.8235, 32.2818) (-17.8109, 32.2852) (-17.794, 32.2891) (-17.7727, 32.293) (-17.7511, 32.2962) (-17.7295, 32.299) (-17.7077, 32.3016) (-17.6859, 32.304) (-17.6641, 32.3063) (-17.6422, 32.3083) (-17.6202, 32.3101) (-17.5982, 32.3115) (-17.5761, 32.3126) (-17.5539, 32.3134) (-17.5316, 32.314) (-17.5093, 32.3143) (-17.4869, 32.3144) (-17.4645, 32.3143) (-17.4421, 32.3141) (-17.4196, 32.3136) (-17.3971, 32.3129) (-17.3745, 32.3121) (-17.3519, 32.311) (-17.3292, 32.3097) (-17.3065, 32.3082) (-17.2838, 32.3066) (-17.2611, 32.3047) (-17.2383, 32.3027) (-17.2154, 32.3005) (-17.1926, 32.2982) (-17.1697, 32.2956) (-17.1468, 32.2929) (-17.1239, 32.29) (-17.1009, 32.287) (-17.0779, 32.2838) (-17.0549, 32.2804) (-17.0319, 32.2768) (-17.0088, 32.2731) (-16.9858, 32.2693) (-16.9627, 32.2652) (-16.9395, 32.2611) (-16.9164, 32.2567) (-16.8933, 32.2522) (-16.8701, 32.2476) (-16.8469, 32.2428) (-16.8237, 32.2378) (-16.8005, 32.2327) (-16.7773, 32.2275) (-16.754, 32.2221) (-16.7308, 32.2165) (-16.7075, 32.2108) (-16.6842, 32.205) (-16.6609, 32.199) (-16.6376, 32.1929) (-16.6143, 32.1866) (-16.591, 32.1802) (-16.5677, 32.1736) (-16.5443, 32.167) (-16.521, 32.1601) (-16.4977, 32.1531) (-16.4743, 32.146) (-16.451, 32.1388) (-16.4276, 32.1314) (-16.4042, 32.1238) (-16.3809, 32.1162) (-16.3575, 32.1084) (-16.3341, 32.1004) (-16.3108, 32.0924) (-16.2874, 32.0842) (-16.2687, 32.0775) (-16.2547, 32.0724) (-16.2453, 32.069) (-16.2406, 32.0673) knots 0 0 0 0 0 0 0.01428571 0.02857143 0.04285714 0.05714286 0.07142857 0.08571429 0.1 0.11428571 0.12857143 0.14285714 0.15714286 0.17142857 0.18571429 0.2 0.21428571 0.22857143 0.24285714 0.25714286 0.27142857 0.28571429 0.3 0.31428571 0.32857143 0.34285714 0.35714286 0.37142857 0.38571429 0.4 0.41428571 0.42857143 0.44285714 0.45714286 0.47142857 0.48571429 0.5 0.51428571 0.52857143 0.54285714 0.55714286 0.57142857 0.58571429 0.6 0.61428571 0.62857143 0.64285714 0.65714286 0.67142857 0.68571429 0.7 0.71428571 0.72857143 0.74285714 0.75714286 0.77142857 0.78571429 0.8 0.81428571 0.82857143 0.84285714 0.85714286 0.87142857 0.88571429 0.9 0.91428571 0.92857143 0.94285714 0.95714286 0.97142857 0.98571429 1 1 1 1 1 1
  arc A29 (-16.1163, 31.4421) -> (-16.2406, 32.0673) centre (-25, 30) ccw
  spline S14 degree 5 poles (-17.5095, 30.637) (-17.5052, 30.6373) (-17.4965, 30.6382) (-17.4837, 30.6399) (-17.4666, 30.6428) (-17.4453, 30.6473) (-17.4242, 30.6526) (-17.4031, 30.6583) (-17.382, 30.6642) (-17.361, 30.6703) (-17.3399, 30.6766) (-17.3189, 30.6831) (-17.298, 30.6899) (-17.277, 30.697) (-17.2562, 30.7044) (-17.2354, 30.7122) (-17.2146, 30.7202) (-17.1939, 30.7285) (-17.1731, 30.7369) (-17.1525, 30.7456) (-17.1318, 30.7544) (-17.1112, 30.7634) (-17.0907, 30.7726) (-17.0702, 30.7821) (-17.0497, 30.7917) (-17.0293, 30.8016) (-17.0089, 30.8116) (-16.9885, 30.8219) (-16.9682, 30.8323) (-16.9479, 30.8429) (-16.9276, 30.8536) (-16.9074, 30.8645) (-16.8873, 30.8756) (-16.8671, 30.8869) (-16.8471, 30.8984) (-16.827, 30.91) (-16.807, 30.9217) (-16.787, 30.9337) (-16.7671, 30.9458) (-16.7472, 30.958) (-16.7274, 30.9704) (-16.7076, 30.983) (-16.6878, 30.9957) (-16.6681, 31.0085) (-16.6485, 31.0215) (-16.6288, 31.0347) (-16.6092, 31.048) (-16.5897, 31.0615) (-16.5702, 31.075) (-16.5508, 31.0888) (-16.5313, 31.1027) (-16.512, 31.1167) (-16.4927, 31.1309) (-16.4734, 31.1452) (-16.4542, 31.1596) (-16.435, 31.1742) (-16.4159, 31.1889) (-16.3968, 31.2037) (-16.3777, 31.2187) (-16.3587, 31.2338) (-16.3398, 31.2491) (-16.3209, 31.2645) (-16.302, 31.28) (-16.2832, 31.2956) (-16.2645, 31.3114) (-16.2458, 31.3273) (-16.2271, 31.3433) (-16.2085, 31.3595) (-16.19, 31.3757) (-16.1715, 31.3921) (-16.153, 31.4087) (-16.1383, 31.422) (-16.1273, 31.432) (-16.12, 31.4387) (-16.1163, 31.4421) knots 0 0 0 0 0 0 0.01428571 0.02857143 0.04285714 0.05714286 0.07142857 0.08571429 0.1 0.11428571 0.12857143 0.14285714 0.15714286 0.17142857 0.18571429 0.2 0.21428571 0.22857143 0.24285714 0.25714286 0.27142857 0.28571429 0.3 0.31428571 0.32857143 0.34285714 0.35714286 0.37142857 0.38571429 0.4 0.41428571 0.42857143 0.44285714 0.45714286 0.47142857 0.48571429 0.5 0.51428571 0.52857143 0.54285714 0.55714286 0.57142857 0.58571429 0.6 0.61428571 0.62857143 0.64285714 0.65714286 0.67142857 0.68571429 0.7 0.71428571 0.72857143 0.74285714 0.75714286 0.77142857 0.78571429 0.8 0.81428571 0.82857143 0.84285714 0.85714286 0.87142857 0.88571429 0.9 0.91428571 0.92857143 0.94285714 0.95714286 0.97142857 0.98571429 1 1 1 1 1 1
  line L17 (-17.5095, 30.637) -> (-17.7948, 30.6123)
  arc A30 (-17.7948, 30.6123) -> (-18.2516, 30.1063) centre (-17.7517, 30.1142) ccw
  arc A31 (-18.2516, 29.8937) -> (-18.2516, 30.1063) centre (-25, 30) ccw
  arc A32 (-18.2516, 29.8937) -> (-17.7948, 29.3877) centre (-17.7517, 29.8858) ccw
  line L18 (-17.7948, 29.3877) -> (-17.5095, 29.363)
  spline S15 degree 5 poles (-17.5095, 29.363) (-17.5052, 29.3627) (-17.4965, 29.3618) (-17.4837, 29.3601) (-17.4666, 29.3572) (-17.4453, 29.3527) (-17.4242, 29.3474) (-17.4031, 29.3417) (-17.382, 29.3358) (-17.361, 29.3297) (-17.3399, 29.3234) (-17.3189, 29.3169) (-17.298, 29.3101) (-17.277, 29.303) (-17.2562, 29.2956) (-17.2354, 29.2878) (-17.2146, 29.2798) (-17.1939, 29.2715) (-17.1731, 29.2631) (-17.1525, 29.2544) (-17.1318, 29.2456) (-17.1112, 29.2366) (-17.0907, 29.2274) (-17.0702, 29.2179) (-17.0497, 29.2083) (-17.0293, 29.1984) (-17.0089, 29.1884) (-16.9885, 29.1781) (-16.9682, 29.1677) (-16.9479, 29.1571) (-16.9276, 29.1464) (-16.9074, 29.1355) (-16.8873, 29.1244) (-16.8671, 29.1131) (-16.8471, 29.1016) (-16.827, 29.09) (-16.807, 29.0783) (-16.787, 29.0663) (-16.7671, 29.0542) (-16.7472, 29.042) (-16.7274, 29.0296) (-16.7076, 29.017) (-16.6878, 29.0043) (-16.6681, 28.9915) (-16.6485, 28.9785) (-16.6288, 28.9653) (-16.6092, 28.952) (-16.5897, 28.9385) (-16.5702, 28.925) (-16.5508, 28.9112) (-16.5313, 28.8973) (-16.512, 28.8833) (-16.4927, 28.8691) (-16.4734, 28.8548) (-16.4542, 28.8404) (-16.435, 28.8258) (-16.4159, 28.8111) (-16.3968, 28.7963) (-16.3777, 28.7813) (-16.3587, 28.7662) (-16.3398, 28.7509) (-16.3209, 28.7355) (-16.302, 28.72) (-16.2832, 28.7044) (-16.2645, 28.6886) (-16.2458, 28.6727) (-16.2271, 28.6567) (-16.2085, 28.6405) (-16.19, 28.6243) (-16.1715, 28.6079) (-16.153, 28.5913) (-16.1383, 28.578) (-16.1273, 28.568) (-16.12, 28.5613) (-16.1163, 28.5579) knots 0 0 0 0 0 0 0.01428571 0.02857143 0.04285714 0.05714286 0.07142857 0.08571429 0.1 0.11428571 0.12857143 0.14285714 0.15714286 0.17142857 0.18571429 0.2 0.21428571 0.22857143 0.24285714 0.25714286 0.27142857 0.28571429 0.3 0.31428571 0.32857143 0.34285714 0.35714286 0.37142857 0.38571429 0.4 0.41428571 0.42857143 0.44285714 0.45714286 0.47142857 0.48571429 0.5 0.51428571 0.52857143 0.54285714 0.55714286 0.57142857 0.58571429 0.6 0.61428571 0.62857143 0.64285714 0.65714286 0.67142857 0.68571429 0.7 0.71428571 0.72857143 0.74285714 0.75714286 0.77142857 0.78571429 0.8 0.81428571 0.82857143 0.84285714 0.85714286 0.87142857 0.88571429 0.9 0.91428571 0.92857143 0.94285714 0.95714286 0.97142857 0.98571429 1 1 1 1 1 1
  arc A33 (-16.2406, 27.9327) -> (-16.1163, 28.5579) centre (-25, 30) ccw
  spline S16 degree 5 poles (-17.8359, 27.722) (-17.8318, 27.7207) (-17.8235, 27.7182) (-17.8109, 27.7148) (-17.794, 27.7109) (-17.7727, 27.707) (-17.7511, 27.7038) (-17.7295, 27.701) (-17.7077, 27.6984) (-17.6859, 27.696) (-17.6641, 27.6937) (-17.6422, 27.6917) (-17.6202, 27.6899) (-17.5982, 27.6885) (-17.5761, 27.6874) (-17.5539, 27.6866) (-17.5316, 27.686) (-17.5093, 27.6857) (-17.4869, 27.6856) (-17.4645, 27.6857) (-17.4421, 27.6859) (-17.4196, 27.6864) (-17.3971, 27.6871) (-17.3745, 27.6879) (-17.3519, 27.689) (-17.3292, 27.6903) (-17.3065, 27.6918) (-17.2838, 27.6934) (-17.2611, 27.6953) (-17.2383, 27.6973) (-17.2154, 27.6995) (-17.1926, 27.7018) (-17.1697, 27.7044) (-17.1468, 27.7071) (-17.1239, 27.71) (-17.1009, 27.713) (-17.0779, 27.7162) (-17.0549, 27.7196) (-17.0319, 27.7232) (-17.0088, 27.7269) (-16.9858, 27.7307) (-16.9627, 27.7348) (-16.9395, 27.7389) (-16.9164, 27.7433) (-16.8933, 27.7478) (-16.8701, 27.7524) (-16.8469, 27.7572) (-16.8237, 27.7622) (-16.8005, 27.7673) (-16.7773, 27.7725) (-16.754, 27.7779) (-16.7308, 27.7835) (-16.7075, 27.7892) (-16.6842, 27.795) (-16.6609, 27.801) (-16.6376, 27.8071) (-16.6143, 27.8134) (-16.591, 27.8198) (-16.5677, 27.8264) (-16.5443, 27.833) (-16.521, 27.8399) (-16.4977, 27.8469) (-16.4743, 27.854) (-16.451, 27.8612) (-16.4276, 27.8686) (-16.4042, 27.8762) (-16.3809, 27.8838) (-16.3575, 27.8916) (-16.3341, 27.8996) (-16.3108, 27.9076) (-16.2874, 27.9158) (-16.2687, 27.9225) (-16.2547, 27.9276) (-16.2453, 27.931) (-16.2406, 27.9327) knots 0 0 0 0 0 0 0.01428571 0.02857143 0.04285714 0.05714286 0.07142857 0.08571429 0.1 0.11428571 0.12857143 0.14285714 0.15714286 0.17142857 0.18571429 0.2 0.21428571 0.22857143 0.24285714 0.25714286 0.27142857 0.28571429 0.3 0.31428571 0.32857143 0.34285714 0.35714286 0.37142857 0.38571429 0.4 0.41428571 0.42857143 0.44285714 0.45714286 0.47142857 0.48571429 0.5 0.51428571 0.52857143 0.54285714 0.55714286 0.57142857 0.58571429 0.6 0.61428571 0.62857143 0.64285714 0.65714286 0.67142857 0.68571429 0.7 0.71428571 0.72857143 0.74285714 0.75714286 0.77142857 0.78571429 0.8 0.81428571 0.82857143 0.84285714 0.85714286 0.87142857 0.88571429 0.9 0.91428571 0.92857143 0.94285714 0.95714286 0.97142857 0.98571429 1 1 1 1 1 1
  line L19 (-17.8359, 27.722) -> (-18.1089, 27.8084)
  arc A34 (-18.1089, 27.8084) -> (-18.7247, 27.5157) centre (-18.2598, 27.3317) ccw
  arc A35 (-18.806, 27.3193) -> (-18.7247, 27.5157) centre (-25, 30) ccw
  arc A36 (-18.806, 27.3193) -> (-18.5776, 26.677) centre (-18.3471, 27.1207) ccw
  line L20 (-18.5776, 26.677) -> (-18.3234, 26.545)
  spline S17 degree 5 poles (-18.3234, 26.545) (-18.3196, 26.543) (-18.3119, 26.5389) (-18.3007, 26.5325) (-18.286, 26.5232) (-18.2681, 26.5109) (-18.2506, 26.4979) (-18.2333, 26.4846) (-18.2161, 26.4711) (-18.199, 26.4574) (-18.182, 26.4435) (-18.165, 26.4295) (-18.1482, 26.4152) (-18.1316, 26.4006) (-18.1152, 26.3858) (-18.0989, 26.3706) (-18.0828, 26.3553) (-18.0668, 26.3397) (-18.0509, 26.324) (-18.0351, 26.3081) (-18.0195, 26.292) (-18.0039, 26.2758) (-17.9884, 26.2594) (-17.9731, 26.2428) (-17.9579, 26.2261) (-17.9427, 26.2092) (-17.9277, 26.1921) (-17.9128, 26.1748) (-17.8981, 26.1574) (-17.8834, 26.1399) (-17.8688, 26.1222) (-17.8543, 26.1044) (-17.8399, 26.0864) (-17.8256, 26.0683) (-17.8114, 26.05) (-17.7974, 26.0316) (-17.7834, 26.0131) (-17.7695, 25.9944) (-17.7557, 25.9756) (-17.742, 25.9567) (-17.7285, 25.9377) (-17.715, 25.9185) (-17.7016, 25.8992) (-17.6883, 25.8798) (-17.6751, 25.8602) (-17.662, 25.8406) (-17.649, 25.8208) (-17.6361, 25.8009) (-17.6233, 25.7808) (-17.6106, 25.7607) (-17.598, 25.7405) (-17.5854, 25.7201) (-17.573, 25.6996) (-17.5607, 25.679) (-17.5484, 25.6583) (-17.5363, 25.6375) (-17.5243, 25.6166) (-17.5123, 25.5956) (-17.5004, 25.5744) (-17.4887, 25.5532) (-17.477, 25.5319) (-17.4654, 25.5104) (-17.454, 25.4889) (-17.4426, 25.4672) (-17.4313, 25.4455) (-17.4201, 25.4237) (-17.409, 25.4017) (-17.398, 25.3797) (-17.3871, 25.3575) (-17.3763, 25.3353) (-17.3655, 25.313) (-17.357, 25.295) (-17.3507, 25.2815) (-17.3465, 25.2725) (-17.3444, 25.268) knots 0 0 0 0 0 0 0.01428571 0.02857143 0.04285714 0.05714286 0.07142857 0.08571429 0.1 0.11428571 0.12857143 0.14285714 0.15714286 0.17142857 0.18571429 0.2 0.21428571 0.22857143 0.24285714 0.25714286 0.27142857 0.28571429 0.3 0.31428571 0.32857143 0.34285714 0.35714286 0.37142857 0.38571429 0.4 0.41428571 0.42857143 0.44285714 0.45714286 0.47142857 0.48571429 0.5 0.51428571 0.52857143 0.54285714 0.55714286 0.57142857 0.58571429 0.6 0.61428571 0.62857143 0.64285714 0.65714286 0.67142857 0.68571429 0.7 0.71428571 0.72857143 0.74285714 0.75714286 0.77142857 0.78571429 0.8 0.81428571 0.82857143 0.84285714 0.85714286 0.87142857 0.88571429 0.9 0.91428571 0.92857143 0.94285714 0.95714286 0.97142857 0.98571429 1 1 1 1 1 1
  arc A37 (-17.6985, 24.738) -> (-17.3444, 25.268) centre (-25, 30) ccw
  spline S18 degree 5 poles (-19.253, 25.1538) (-19.2497, 25.151) (-19.243, 25.1455) (-19.2327, 25.1376) (-19.2186, 25.1276) (-19.2003, 25.1158) (-19.1816, 25.1046) (-19.1627, 25.0937) (-19.1436, 25.083) (-19.1244, 25.0724) (-19.1051, 25.062) (-19.0856, 25.0517) (-19.066, 25.0417) (-19.0462, 25.0319) (-19.0262, 25.0224) (-19.006, 25.0132) (-18.9856, 25.0041) (-18.9651, 24.9953) (-18.9445, 24.9867) (-18.9238, 24.9782) (-18.9029, 24.9698) (-18.882, 24.9616) (-18.8609, 24.9536) (-18.8397, 24.9458) (-18.8184, 24.9381) (-18.797, 24.9306) (-18.7755, 24.9233) (-18.7539, 24.9162) (-18.7321, 24.9091) (-18.7103, 24.9023) (-18.6884, 24.8956) (-18.6664, 24.889) (-18.6443, 24.8826) (-18.6221, 24.8763) (-18.5998, 24.8702) (-18.5774, 24.8643) (-18.5549, 24.8584) (-18.5324, 24.8528) (-18.5097, 24.8472) (-18.487, 24.8418) (-18.4642, 24.8366) (-18.4413, 24.8314) (-18.4184, 24.8265) (-18.3953, 24.8216) (-18.3722, 24.8169) (-18.349, 24.8123) (-18.3258, 24.8079) (-18.3025, 24.8036) (-18.2791, 24.7994) (-18.2556, 24.7954) (-18.2321, 24.7915) (-18.2084, 24.7877) (-18.1848, 24.784) (-18.161, 24.7805) (-18.1372, 24.7771) (-18.1134, 24.7739) (-18.0894, 24.7708) (-18.0654, 24.7678) (-18.0414, 24.7649) (-18.0172, 24.7622) (-17.9931, 24.7595) (-17.9688, 24.7571) (-17.9445, 24.7547) (-17.9202, 24.7525) (-17.8958, 24.7503) (-17.8713, 24.7484) (-17.8468, 24.7465) (-17.8222, 24.7448) (-17.7976, 24.7432) (-17.7729, 24.7417) (-17.7482, 24.7403) (-17.7283, 24.7393) (-17.7135, 24.7386) (-17.7035, 24.7382) (-17.6985, 24.738) knots 0 0 0 0 0 0 0.01428571 0.02857143 0.04285714 0.05714286 0.07142857 0.08571429 0.1 0.11428571 0.12857143 0.14285714 0.15714286 0.17142857 0.18571429 0.2 0.21428571 0.22857143 0.24285714 0.25714286 0.27142857 0.28571429 0.3 0.31428571 0.32857143 0.34285714 0.35714286 0.37142857 0.38571429 0.4 0.41428571 0.42857143 0.44285714 0.45714286 0.47142857 0.48571429 0.5 0.51428571 0.52857143 0.54285714 0.55714286 0.57142857 0.58571429 0.6 0.61428571 0.62857143 0.64285714 0.65714286 0.67142857 0.68571429 0.7 0.71428571 0.72857143 0.74285714 0.75714286 0.77142857 0.78571429 0.8 0.81428571 0.82857143 0.84285714 0.85714286 0.87142857 0.88571429 0.9 0.91428571 0.92857143 0.94285714 0.95714286 0.97142857 0.98571429 1 1 1 1 1 1
  line L21 (-19.253, 25.1538) -> (-19.4722, 25.3381)
  arc A38 (-19.4722, 25.3381) -> (-20.153, 25.3033) centre (-19.794, 24.9554) ccw
  arc A39 (-20.3033, 25.153) -> (-20.153, 25.3033) centre (-25, 30) ccw
  arc A40 (-20.3033, 25.153) -> (-20.3381, 24.4722) centre (-19.9554, 24.794) ccw
  line L22 (-20.3381, 24.4722) -> (-20.1538, 24.253)
  spline S19 degree 5 poles (-20.1538, 24.253) (-20.151, 24.2497) (-20.1455, 24.243) (-20.1376, 24.2327) (-20.1276, 24.2186) (-20.1158, 24.2003) (-20.1046, 24.1816) (-20.0937, 24.1627) (-20.083, 24.1436) (-20.0724, 24.1244) (-20.062, 24.1051) (-20.0517, 24.0856) (-20.0417, 24.066) (-20.0319, 24.0462) (-20.0224, 24.0262) (-20.0132, 24.006) (-20.0041, 23.9856) (-19.9953, 23.9651) (-19.9867, 23.9445) (-19.9782, 23.9238) (-19.9698, 23.9029) (-19.9616, 23.882) (-19.9536, 23.8609) (-19.9458, 23.8397) (-19.9381, 23.8184) (-19.9306, 23.797) (-19.9233, 23.7755) (-19.9162, 23.7539) (-19.9091, 23.7321) (-19.9023, 23.7103) (-19.8956, 23.6884) (-19.889, 23.6664) (-19.8826, 23.6443) (-19.8763, 23.6221) (-19.8702, 23.5998) (-19.8643, 23.5774) (-19.8584, 23.5549) (-19.8528, 23.5324) (-19.8472, 23.5097) (-19.8418, 23.487) (-19.8366, 23.4642) (-19.8314, 23.4413) (-19.8265, 23.4184) (-19.8216, 23.3953) (-19.8169, 23.3722) (-19.8123, 23.349) (-19.8079, 23.3258) (-19.8036, 23.3025) (-19.7994, 23.2791) (-19.7954, 23.2556) (-19.7915, 23.2321) (-19.7877, 23.2084) (-19.784, 23.1848) (-19.7805, 23.161) (-19.7771, 23.1372) (-19.7739, 23.1134) (-19.7708, 23.0894) (-19.7678, 23.0654) (-19.7649, 23.0414) (-19.7622, 23.0172) (-19.7595, 22.9931) (-19.7571, 22.9688) (-19.7547, 22.9445) (-19.7525, 22.9202) (-19.7503, 22.8958) (-19.7484, 22.8713) (-19.7465, 22.8468) (-19.7448, 22.8222) (-19.7432, 22.7976) (-19.7417, 22.7729) (-19.7403, 22.7482) (-19.7393, 22.7283) (-19.7386, 22.7135) (-19.7382, 22.7035) (-19.738, 22.6985) knots 0 0 0 0 0 0 0.01428571 0.02857143 0.04285714 0.05714286 0.07142857 0.08571429 0.1 0.11428571 0.12857143 0.14285714 0.15714286 0.17142857 0.18571429 0.2 0.21428571 0.22857143 0.24285714 0.25714286 0.27142857 0.28571429 0.3 0.31428571 0.32857143 0.34285714 0.35714286 0.37142857 0.38571429 0.4 0.41428571 0.42857143 0.44285714 0.45714286 0.47142857 0.48571429 0.5 0.51428571 0.52857143 0.54285714 0.55714286 0.57142857 0.58571429 0.6 0.61428571 0.62857143 0.64285714 0.65714286 0.67142857 0.68571429 0.7 0.71428571 0.72857143 0.74285714 0.75714286 0.77142857 0.78571429 0.8 0.81428571 0.82857143 0.84285714 0.85714286 0.87142857 0.88571429 0.9 0.91428571 0.92857143 0.94285714 0.95714286 0.97142857 0.98571429 1 1 1 1 1 1
  arc A41 (-20.268, 22.3444) -> (-19.738, 22.6985) centre (-25, 30) ccw